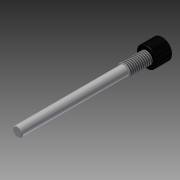
# Autodesk Inventor part: Rod Bolt Side
Saved by Autodesk Inventor 2013 (Build 170138000, 138)
## iProperties
Created: 2013-05-10
Part Number: Rod Bolt Side
Material: Generic
Document SubType Name: Modeling
Designer: grtstudent
Density: 1 g/cm^3
Author: grtstudent
Autodesk Inventor part; units mm, degrees
ref_plane "YZ Plane" through (0, 0, 0) normal (1, 0, 0) x (0, 1, 0)
ref_plane "XZ Plane" through (0, 0, 0) normal (0, 1, 0) x (-1, 0, 0)
ref_plane "XY Plane" through (0, 0, 0) normal (0, 0, 1) x (1, 0, 0)
sketch "Sketch1" plane through (0, 0, 0) normal (0, 0, 1) x (1, 0, 0)
  circle A0 centre (0, 0) radius 3.9688
  dimension "d0" = 7.9375
  constraints: 1 centre point, 1 coincident
  measures "d0" diameter of A0
extrude "Extrusion1" add sketch "Sketch1" along normal blind 6.35
sketch "Sketch2" plane through (0, 0, 6.35) normal (0, 0, 1) x (1, 0, 0)
  circle A0 centre (0, 0) radius 3.9688 projected
  circle A1 centre (0, 0) radius 2.413
  dimension "d4" = 4.826
  constraints: 1 centre point, 1 coincident
  measures "d4" diameter of A1
extrude "Extrusion2" add sketch "Sketch2" along normal blind 8.89 contours A1
thread "Thread1" size "10-32 UNF" class "2A" standard "ANSI Unified Screw Threads" full length
sketch "Sketch3" plane through (0, 0, 15.24) normal (0, 0, 1) x (1, 0, 0)
  circle A0 centre (0, 0) radius 2.413 projected
  circle A1 centre (0, 0) radius 1.8986
  dimension "d17" = 3.7973
  constraints: 1 centre point, 1 coincident
  measures "d17" diameter of A1
extrude "Extrusion3" add sketch "Sketch3" along normal blind 41.91 contours A1
sketch "Sketch4" plane through (0, 0, 0) normal (0, 0, -1) x (-1, 0, 0)
  circle A0 centre (0, 0) radius 3.9688 projected
  line L0 (-2.2914, 0) -> (-1.1457, 1.9844)
  line L1 (-1.1457, 1.9844) -> (1.1457, 1.9844)
  line L2 (1.1457, 1.9844) -> (2.2914, 0)
  line L3 (2.2914, 0) -> (1.1457, -1.9844)
  line L4 (1.1457, -1.9844) -> (-1.1457, -1.9844)
  line L5 (-1.1457, -1.9844) -> (-2.2914, 0)
  dimension "d23" = 3.9688
  constraints: 12 end point, 1 coincident, 1 horizontal, 13 other
  measures "d23" distance between parallel lines of L4 L1
extrude "Extrusion4" cut sketch "Sketch4" against normal blind 3.175 contours L0 L1 L2 L3 L4 L5
chamfer "Chamfer1" distance 0.254 angle 45 3 edges at (-3.9688, 0, 0) (-3.9688, 0, 6.35) (-1.8986, 0, 57.15)
chamfer "Chamfer2" distance 0.127 angle 45 1 edges at (-2.413, 0, 15.24)
body "Solid1"
